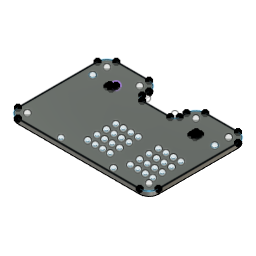
合页连接板-方案二-改 v3 (Autodesk Fusion 360 design; units mm, degrees)
Autodesk Fusion 360 part; units mm, degrees
sketch "草图1" plane through (0, 0, 0) normal (0, 0, 1) x (1, 0, 0)
  line L0 (75, -52.5) -> (-75, -52.5)
  line L1 (-75, -52.5) -> (-75, 52.5)
  line L2 (-75, 52.5) -> (75, 52.5)
  line L3 (75, 52.5) -> (75, -52.5)
  line L4 (75, -52.5) -> (-75, 52.5) construction
  line L5 (-75, -52.5) -> (75, 52.5) construction
  line L6 (-75, 27.5) -> (75, 27.5) construction
  line L7 (0, 52.5) -> (0, 0) construction
  line L8 (-35, 52.5) -> (-35, 27.5) construction
  line L9 (35, 52.5) -> (35, 27.5) construction
  circle A0 centre (-65.15, 27.5) radius 2.65
  circle A1 centre (65.15, 27.5) radius 2.65
  line L10 (-65.15, 30.15) -> (-65.15, 24.85) construction
  line L11 (65.15, 24.85) -> (65.15, 30.15) construction
  line L12 (65.15, 24.85) -> (-65.15, 24.85)
  line L13 (-65.15, 30.15) -> (65.15, 30.15)
  circle A2 centre (-46.85, 27.5) radius 2.65
  circle A3 centre (-42.85, 27.5) radius 2.65
  circle A4 centre (42.85, 27.5) radius 2.65
  circle A5 centre (46.85, 27.5) radius 2.65
  line L14 (-75, -5.5) -> (75, -5.5) construction
  line L15 (-75, -35.5) -> (75, -35.5) construction
  line L16 (-75, -47.5) -> (75, -47.5) construction
  circle A6 centre (-24, -47.5) radius 1.525
  circle A7 centre (32, -47.5) radius 1.525
  line L17 (-75, -25.5) -> (75, -25.5) construction
  line L18 (-75, -15.5) -> (75, -15.5) construction
  line L19 (62, -35.5) -> (62, -5.5) construction
  line L20 (-7.5, -35.5) -> (-7.5, -5.5) construction
  line L21 (0.5, -35.5) -> (0.5, -5.5) construction
  line L22 (8.5, -35.5) -> (8.5, -5.5) construction
  line L23 (16.5, -35.5) -> (16.5, -5.5) construction
  line L24 (38, -35.5) -> (38, -5.5) construction
  line L25 (46, -35.5) -> (46, -5.5) construction
  line L26 (54, -35.5) -> (54, -5.5) construction
  circle A8 centre (62, -5.5) radius 1.5
  circle A9 centre (62, -15.5) radius 1.5
  circle A10 centre (62, -25.5) radius 1.5
  circle A11 centre (62, -35.5) radius 1.5
  circle A12 centre (54, -5.5) radius 1.5
  circle A13 centre (54, -15.5) radius 1.5
  circle A14 centre (54, -25.5) radius 1.5
  circle A15 centre (54, -35.5) radius 1.5
  circle A16 centre (46, -5.5) radius 1.5
  circle A17 centre (46, -15.5) radius 1.5
  circle A18 centre (46, -25.5) radius 1.5
  circle A19 centre (38, -25.5) radius 1.5
  circle A20 centre (38, -5.5) radius 1.5
  circle A21 centre (38, -15.5) radius 1.5
  circle A22 centre (38, -35.5) radius 1.5
  circle A23 centre (46, -35.5) radius 1.5
  circle A24 centre (16.5, -5.5) radius 1.5
  circle A25 centre (8.5, -5.5) radius 1.5
  circle A26 centre (0.5, -5.5) radius 1.5
  circle A27 centre (-7.5, -5.5) radius 1.5
  circle A28 centre (16.5, -15.5) radius 1.5
  circle A29 centre (8.5, -15.5) radius 1.5
  circle A30 centre (0.5, -15.5) radius 1.5
  circle A31 centre (-7.5, -15.5) radius 1.5
  circle A32 centre (-7.5, -25.5) radius 1.5
  circle A33 centre (0.5, -25.5) radius 1.5
  circle A34 centre (8.5, -25.5) radius 1.5
  circle A35 centre (16.5, -25.5) radius 1.5
  circle A36 centre (16.5, -35.5) radius 1.5
  circle A37 centre (8.5, -35.5) radius 1.5
  circle A38 centre (0.5, -35.5) radius 1.5
  circle A39 centre (-7.5, -35.5) radius 1.5
  line L27 (-20, 52.5) -> (-20, 30.15)
  line L28 (20, 52.5) -> (20, 30.15)
  point P0 (-65.15, 27.5)
  point P1 (65.15, 27.5)
  point P2 (-44.85, 27.5)
  point P3 (44.85, 27.5)
  point P4 (0, 27.5)
  point P5 (-46.85, 27.5)
  point P6 (-42.85, 27.5)
  point P7 (42.85, 27.5)
  point P8 (46.85, 27.5)
  point P9 (32, -47.5)
  point P10 (-24, -47.5)
  point P11 (0.5, -35.5)
  point P12 (8.5, -35.5)
  point P13 (16.5, -35.5)
  point P14 (-7.5, -25.5)
  point P15 (-7.5, -5.5)
  point P16 (-7.5, -35.5)
  point P17 (-7.5, -15.5)
  point P18 (-7.5, -25.5)
  point P19 (62, -35.5)
  point P20 (62, -25.5)
  point P21 (62, -15.5)
  point P22 (62, -5.5)
  point P23 (54, -35.5)
  point P24 (46, -35.5)
  point P25 (38, -35.5)
  point P26 (0.5, -25.5)
  point P27 (0.5, -15.5)
  point P28 (0.5, -5.5)
  point P29 (8.5, -25.5)
  point P30 (8.5, -15.5)
  point P31 (8.5, -5.5)
  point P32 (16.5, -25.5)
  point P33 (16.5, -15.5)
  point P34 (16.5, -5.5)
  point P35 (38, -25.5)
  point P36 (38, -15.5)
  point P37 (38, -5.5)
  point P38 (46, -25.5)
  point P39 (46, -15.5)
  point P40 (46, -5.5)
  point P41 (54, -25.5)
  point P42 (54, -15.5)
  point P43 (54, -5.5)
  dimension "d1" = 150
  dimension "d2" = 105
  dimension "d3" = 25
  dimension "d4" = 20.3
  dimension "d5" = 20.3
  dimension "d6" = 9.85
  dimension "d7" = 44.85
  dimension "d8" = 9.85
  dimension "d9" = 44.85
  dimension "d10" = 40
  dimension "d11" = 40
  dimension "d12" = 70
  dimension "d13" = 5.3
  dimension "d14" = 5.3
  dimension "d15" = 2
  dimension "d16" = 2
  dimension "d17" = 2
  dimension "d18" = 2
  dimension "d20" = 30
  dimension "d24" = 56
  dimension "d25" = 3.05
  dimension "d26" = 3.05
  dimension "d27" = 10
  dimension "d28" = 10
  dimension "d29" = 10
  dimension "d30" = 13
  dimension "d35" = 8
  dimension "d36" = 16
  dimension "d37" = 24
  dimension "d38" = 3
  dimension "d39" = 3
  dimension "d40" = 3
  dimension "d41" = 3
  dimension "d42" = 3
  dimension "d43" = 3
  dimension "d44" = 3
  dimension "d45" = 3
  dimension "d46" = 3
  dimension "d47" = 3
  dimension "d48" = 3
  dimension "d49" = 3
  dimension "d50" = 3
  dimension "d51" = 3
  dimension "d52" = 3
  dimension "d53" = 3
  dimension "d54" = 3
  dimension "d55" = 3
  dimension "d56" = 3
  dimension "d57" = 3
  dimension "d58" = 3
  dimension "d59" = 3
  dimension "d60" = 3
  dimension "d61" = 3
  dimension "d62" = 3
  dimension "d63" = 3
  dimension "d64" = 3
  dimension "d65" = 3
  dimension "d66" = 3
  dimension "d67" = 3
  dimension "d68" = 3
  dimension "d69" = 3
  dimension "d72" = 21.5
  dimension "d73" = 21.5
  dimension "d74" = 8
  dimension "d75" = 8
  dimension "d76" = 8
  dimension "d77" = 20
  dimension "d84" = 51
  dimension "d87" = 5
  dimension "d88" = 12
  constraint horizontal L0
  constraint perpendicular L0 L1
  constraint parallel L0 L2
  constraint parallel L1 L3
  constraint coincident L4 L7.end
  constraint coincident L5 L7.end
  constraint coincident L7.end origin
  constraint coincident L1 L6.start
  constraint coincident L3 L6.end
  constraint perpendicular L3 L6
  constraint coincident L6 P0
  constraint coincident L6 P1
  constraint coincident L6 P2
  constraint coincident L6 P3
  constraint midpoint L2 L7.start
  constraint symmetric P2 P3 L7
  constraint midpoint L6 P4
  constraint coincident L2 L8.start
  constraint coincident L6 L8.end
  constraint perpendicular L6 L8
  constraint coincident L2 L9.start
  constraint coincident L6 L9.end
  constraint perpendicular L6 L9
  constraint coincident P0 A0.centre
  constraint coincident P1 A1.centre
  constraint coincident A0 L10.start
  constraint coincident A0 L10.end
  constraint perpendicular L6 L10
  constraint coincident A1 L11.start
  constraint coincident A1 L11.end
  constraint perpendicular L6 L11
  constraint tangent A0 L12
  constraint coincident L6 P5
  constraint coincident L6 P6
  constraint coincident L6 P7
  constraint coincident L6 P8
  constraint coincident P5 A2.centre
  constraint tangent L12 A2
  constraint coincident P6 A3.centre
  constraint tangent L12 A3
  constraint coincident P7 A4.centre
  constraint tangent L12 A4
  constraint coincident P8 A5.centre
  constraint tangent L12 A5
  constraint coincident L1 L14.start
  constraint coincident L3 L14.end
  constraint perpendicular L3 L14
  constraint coincident L1 L15.start
  constraint coincident L3 L15.end
  constraint perpendicular L3 L15
  constraint coincident L1 L16.start
  constraint coincident L3 L16.end
  constraint perpendicular L3 L16
  constraint coincident L16 P9
  constraint coincident L16 P10
  constraint coincident P10 A6.centre
  constraint coincident P9 A7.centre
  constraint coincident L1 L17.start
  constraint coincident L3 L17.end
  constraint perpendicular L3 L17
  constraint coincident L1 L18.start
  constraint coincident L3 L18.end
  constraint perpendicular L3 L18
  constraint coincident L15 P19
  constraint coincident L14 P22
  constraint perpendicular L14 L19
  constraint coincident L15 P16
  constraint coincident L14 P15
  constraint perpendicular L14 L20
  constraint coincident L15 P11
  constraint coincident L15 P12
  constraint coincident L15 P13
  constraint coincident L20 P18
  constraint coincident L17 P18
  constraint coincident P15 L20.end
  constraint coincident P16 L20.start
  constraint coincident L18 P17
  constraint coincident L20 P17
  constraint coincident P18 P14
  constraint coincident P19 L19.start
  constraint coincident L19 P20
  constraint coincident L17 P20
  constraint coincident L19 P21
  constraint coincident L18 P21
  constraint coincident P22 L19.end
  constraint coincident L15 P23
  constraint coincident L15 P24
  constraint coincident L15 P25
  constraint coincident L17 P26
  constraint coincident L18 P27
  constraint coincident L14 P28
  constraint coincident L17 P29
  constraint coincident L18 P30
  constraint coincident L14 P31
  constraint coincident L17 P32
  constraint coincident L18 P33
  constraint coincident L14 P34
  constraint coincident L17 P35
  constraint coincident L18 P36
  constraint coincident L14 P37
  constraint coincident L17 P38
  constraint coincident L18 P39
  constraint coincident L14 P40
  constraint coincident L17 P41
  constraint coincident L18 P42
  constraint coincident L14 P43
  constraint coincident P11 L21.start
  constraint coincident P28 L21.end
  constraint perpendicular L14 L21
  constraint coincident P12 L22.start
  constraint coincident P31 L22.end
  constraint perpendicular L14 L22
  constraint coincident P13 L23.start
  constraint coincident P34 L23.end
  constraint perpendicular L14 L23
  constraint coincident P25 L24.start
  constraint coincident P37 L24.end
  constraint perpendicular L14 L24
  constraint coincident P24 L25.start
  constraint coincident P40 L25.end
  constraint perpendicular L14 L25
  constraint coincident P23 L26.start
  constraint coincident P43 L26.end
  constraint perpendicular L14 L26
  constraint coincident P21 A9.centre
  constraint coincident P20 A10.centre
  constraint coincident P42 A13.centre
  constraint coincident P41 A14.centre
  constraint coincident P39 A17.centre
  constraint coincident P38 A18.centre
  constraint coincident P35 A19.centre
  constraint coincident P36 A21.centre
  constraint coincident P33 A28.centre
  constraint coincident P30 A29.centre
  constraint coincident P27 A30.centre
  constraint coincident P17 A31.centre
  constraint coincident P26 A33.centre
  constraint coincident P29 A34.centre
  constraint coincident P32 A35.centre
  constraint coincident P42 L26
  constraint coincident L26 P41
  constraint coincident P38 L25
  constraint coincident P39 L25
  constraint coincident P36 L24
  constraint coincident L24 P35
  constraint coincident L23 P33
  constraint coincident P30 L22
  constraint coincident L22 P29
  constraint coincident L21 P26
  constraint coincident P27 L21
  constraint coincident L2 L27.start
  constraint coincident L13 L27.end
  constraint perpendicular L13 L27
  constraint coincident L2 L28.start
  constraint coincident L13 L28.end
  constraint perpendicular L13 L28
  measures "d1" distance of L1.end L2.end
  measures "d2" distance of L0.end L1.end
  measures "d3" distance of L2 L6
  measures "d4" distance of P0 P2
  measures "d5" distance of P1 P3
  measures "d6" distance of L1 P0
  measures "d7" distance of P2 P4
  measures "d8" distance of L6.end P1
  measures "d9" distance of P3 P4
  measures "d10" distance of L1 L8
  measures "d11" distance of L3 L9
  measures "d12" distance of L8.end L9.end
  measures "d13" diameter of A0
  measures "d14" diameter of A1
  measures "d15" distance of P2 P5
  measures "d16" distance of P2 P6
  measures "d17" distance of P3 P7
  measures "d18" distance of P3 P8
  measures "d20" distance of L14 L15
  measures "d24" distance of P9 P10
  measures "d25" diameter of A6
  measures "d26" diameter of A7
  measures "d27" distance of L14 L18
  measures "d28" distance of L15 L17
  measures "d29" distance of L17 L18
  measures "d30" distance of L3 L19
  measures "d35" distance of P19 P23
  measures "d36" distance of P19 P24
  measures "d37" distance of L19 P25
  measures "d38" diameter of A8
  measures "d39" diameter of A9
  measures "d40" diameter of A10
  measures "d41" diameter of A11
  measures "d42" diameter of A12
  measures "d43" diameter of A13
  measures "d44" diameter of A14
  measures "d45" diameter of A15
  measures "d46" diameter of A16
  measures "d47" diameter of A17
  measures "d48" diameter of A18
  measures "d49" diameter of A19
  measures "d50" diameter of A20
  measures "d51" diameter of A21
  measures "d52" diameter of A22
  measures "d53" diameter of A23
  measures "d54" diameter of A24
  measures "d55" diameter of A25
  measures "d56" diameter of A26
  measures "d57" diameter of A27
  measures "d58" diameter of A28
  measures "d59" diameter of A29
  measures "d60" diameter of A30
  measures "d61" diameter of A31
  measures "d62" diameter of A32
  measures "d63" diameter of A33
  measures "d64" diameter of A34
  measures "d65" diameter of A35
  measures "d66" diameter of A36
  measures "d67" diameter of A37
  measures "d68" diameter of A38
  measures "d69" diameter of A39
  measures "d72" distance of P35 P32
  measures "d73" distance of P33 P36
  measures "d74" distance of L22 L23
  measures "d75" distance of L21 L22
  measures "d76" distance of L20 L21
  measures "d77" distance of L7 L27
  measures "d84" distance of L1 P10
  measures "d87" distance of L0 L16
  measures "d88" distance of L15 L16
extrude "拉伸4" add sketch "草图1" along normal blind 5 contours L0 L1 L2 L3 A0 A1 L12 L13 L27 L28 | L12 L13 A3 A4 | A1 L12 L13 A5 | A0 L12 L13 A2
fillet "圆角3" radius 10 6 edges at (-75, 52.5, 2.5) (-75, -52.5, 2.5) (75, -52.5, 2.5) (-20, 52.5, 2.5) (75, 52.5, 2.5) (20, 52.5, 2.5)
fillet "圆角4" radius 5 2 edges at (-20, 30.15, 2.5) (20, 30.15, 2.5)
sketch "草图2" plane through (0, 0, 5) normal (0, 0, 1) x (-1, 0, 0)
  arc A0 (-30, -52.5) -> (-20, -42.5) centre (-30, -42.5) ccw
  line L0 (-20, -42.5) -> (-20, -35.15)
  arc A1 (-15, -30.15) -> (-20, -35.15) centre (-15, -35.15) ccw
  line L1 (-15, -30.15) -> (15, -30.15)
  arc A2 (20, -35.15) -> (15, -30.15) centre (15, -35.15) ccw
  line L2 (20, -35.15) -> (20, -42.5)
  arc A3 (20, -42.5) -> (30, -52.5) centre (30, -42.5) ccw
  line L3 (30, -52.5) -> (65, -52.5)
  arc A4 (65, -52.5) -> (75, -42.5) centre (65, -42.5) ccw
  line L4 (75, -42.5) -> (75, 42.5)
  arc A5 (75, 42.5) -> (65, 52.5) centre (65, 42.5) ccw
  line L5 (65, 52.5) -> (-65, 52.5)
  arc A6 (-65, 52.5) -> (-75, 42.5) centre (-65, 42.5) ccw
  line L6 (-75, 42.5) -> (-75, -42.5)
  arc A7 (-75, -42.5) -> (-65, -52.5) centre (-65, -42.5) ccw
  line L7 (-65, -52.5) -> (-30, -52.5)
  circle A8 centre (7.5, 15.5) radius 1.5
  circle A9 centre (7.5, 25.5) radius 1.5
  circle A10 centre (-8.5, 25.5) radius 1.5
  circle A11 centre (-0.5, 25.5) radius 1.5
  arc A12 (46.85, -30.15) -> (46.85, -24.85) centre (46.85, -27.5) ccw
  line L8 (46.85, -30.15) -> (42.85, -30.15)
  arc A13 (42.85, -24.85) -> (42.85, -30.15) centre (42.85, -27.5) ccw
  line L9 (42.85, -24.85) -> (46.85, -24.85)
  circle A14 centre (65.15, -27.5) radius 2.65
  arc A15 (-42.85, -30.15) -> (-42.85, -24.85) centre (-42.85, -27.5) ccw
  line L10 (-42.85, -30.15) -> (-46.85, -30.15)
  arc A16 (-46.85, -24.85) -> (-46.85, -30.15) centre (-46.85, -27.5) ccw
  line L11 (-46.85, -24.85) -> (-42.85, -24.85)
  circle A17 centre (-0.5, 35.5) radius 1.5
  circle A18 centre (-16.5, 25.5) radius 1.5
  circle A19 centre (-16.5, 35.5) radius 1.5
  circle A20 centre (-8.5, 35.5) radius 1.5
  circle A21 centre (-65.15, -27.5) radius 2.65
  circle A22 centre (7.5, 35.5) radius 1.5
  circle A23 centre (-0.5, 15.5) radius 1.5
  circle A24 centre (-8.5, 15.5) radius 1.5
  circle A25 centre (-16.5, 15.5) radius 1.5
  circle A26 centre (7.5, 5.5) radius 1.5
  circle A27 centre (-0.5, 5.5) radius 1.5
  circle A28 centre (-8.5, 5.5) radius 1.5
  circle A29 centre (-16.5, 5.5) radius 1.5
  circle A30 centre (-46, 35.5) radius 1.5
  circle A31 centre (-38, 35.5) radius 1.5
  circle A32 centre (-38, 15.5) radius 1.5
  circle A33 centre (-38, 5.5) radius 1.5
  circle A34 centre (-38, 25.5) radius 1.5
  circle A35 centre (-46, 25.5) radius 1.5
  circle A36 centre (-46, 15.5) radius 1.5
  circle A37 centre (-46, 5.5) radius 1.5
  circle A38 centre (-54, 35.5) radius 1.5
  circle A39 centre (-54, 25.5) radius 1.5
  circle A40 centre (-54, 15.5) radius 1.5
  circle A41 centre (-54, 5.5) radius 1.5
  circle A42 centre (-62, 35.5) radius 1.5
  circle A43 centre (-62, 25.5) radius 1.5
  circle A44 centre (-62, 15.5) radius 1.5
  circle A45 centre (-62, 5.5) radius 1.5
  circle A46 centre (-32, 47.5) radius 1.525
  circle A47 centre (24, 47.5) radius 1.525
  circle A48 centre (-32, 47.5) radius 1.525
  circle A49 centre (24, 47.5) radius 1.525
  circle A50 centre (7.5, 35.5) radius 1.5
  circle A51 centre (-0.5, 35.5) radius 1.5
  circle A52 centre (-8.5, 35.5) radius 1.5
  circle A53 centre (-16.5, 35.5) radius 1.5
  circle A54 centre (-38, 35.5) radius 1.5
  circle A55 centre (-46, 35.5) radius 1.5
  circle A56 centre (-54, 35.5) radius 1.5
  circle A57 centre (-62, 35.5) radius 1.5
  circle A58 centre (-62, 25.5) radius 1.5
  circle A59 centre (-54, 25.5) radius 1.5
  circle A60 centre (-46, 25.5) radius 1.5
  circle A61 centre (-38, 25.5) radius 1.5
  circle A62 centre (-16.5, 25.5) radius 1.5
  circle A63 centre (-8.5, 25.5) radius 1.5
  circle A64 centre (-0.5, 25.5) radius 1.5
  circle A65 centre (7.5, 25.5) radius 1.5
  circle A66 centre (7.5, 15.5) radius 1.5
  circle A67 centre (-0.5, 15.5) radius 1.5
  circle A68 centre (-8.5, 15.5) radius 1.5
  circle A69 centre (-16.5, 15.5) radius 1.5
  circle A70 centre (-38, 15.5) radius 1.5
  circle A71 centre (-46, 15.5) radius 1.5
  circle A72 centre (-54, 15.5) radius 1.5
  circle A73 centre (-62, 15.5) radius 1.5
  circle A74 centre (-62, 5.5) radius 1.5
  circle A75 centre (-54, 5.5) radius 1.5
  circle A76 centre (-46, 5.5) radius 1.5
  circle A77 centre (-38, 5.5) radius 1.5
  circle A78 centre (-16.5, 5.5) radius 1.5
  circle A79 centre (-8.5, 5.5) radius 1.5
  circle A80 centre (-0.5, 5.5) radius 1.5
  circle A81 centre (7.5, 5.5) radius 1.5
  circle A82 centre (65.15, -27.5) radius 2.65
  circle A83 centre (-65.15, -27.5) radius 2.65
  line L12 (-46.85, -24.85) -> (-42.85, -24.85)
  line L13 (-46.85, -30.15) -> (-42.85, -30.15)
  arc A84 (-46.85, -24.85) -> (-46.85, -30.15) centre (-46.85, -27.5) ccw
  arc A85 (-42.85, -30.15) -> (-42.85, -24.85) centre (-42.85, -27.5) ccw
  arc A86 (42.85, -24.85) -> (42.85, -30.15) centre (42.85, -27.5) ccw
  arc A87 (46.85, -30.15) -> (46.85, -24.85) centre (46.85, -27.5) ccw
  line L14 (42.85, -24.85) -> (46.85, -24.85)
  line L15 (42.85, -30.15) -> (46.85, -30.15)
  line L16 (-65, -52.5) -> (-30, -52.5)
  line L17 (-20, -42.5) -> (-20, -35.15)
  line L18 (20, -35.15) -> (20, -42.5)
  line L19 (15, -30.15) -> (-15, -30.15)
  line L20 (30, -52.5) -> (65, -52.5)
  line L21 (-75, -42.5) -> (-75, 42.5)
  line L22 (-65, 52.5) -> (65, 52.5)
  line L23 (75, 42.5) -> (75, -42.5)
  arc A88 (-65, 52.5) -> (-75, 42.5) centre (-65, 42.5) ccw
  arc A89 (75, 42.5) -> (65, 52.5) centre (65, 42.5) ccw
  arc A90 (65, -52.5) -> (75, -42.5) centre (65, -42.5) ccw
  arc A91 (20, -42.5) -> (30, -52.5) centre (30, -42.5) ccw
  arc A92 (20, -35.15) -> (15, -30.15) centre (15, -35.15) ccw
  arc A93 (-15, -30.15) -> (-20, -35.15) centre (-15, -35.15) ccw
  arc A94 (-30, -52.5) -> (-20, -42.5) centre (-30, -42.5) ccw
  arc A95 (-75, -42.5) -> (-65, -52.5) centre (-65, -42.5) ccw
  dimension "d95" = 21.5
  constraint concentric A46 A48
  constraint concentric A47 A49
  constraint concentric A22 A50
  constraint concentric A17 A51
  constraint concentric A20 A52
  constraint concentric A19 A53
  constraint concentric A31 A54
  constraint concentric A30 A55
  constraint concentric A38 A56
  constraint concentric A42 A57
  constraint concentric A43 A58
  constraint concentric A39 A59
  constraint concentric A35 A60
  constraint concentric A34 A61
  constraint concentric A18 A62
  constraint concentric A10 A63
  constraint concentric A11 A64
  constraint concentric A9 A65
  constraint concentric A8 A66
  constraint concentric A23 A67
  constraint concentric A24 A68
  constraint concentric A25 A69
  constraint concentric A32 A70
  constraint concentric A36 A71
  constraint concentric A40 A72
  constraint concentric A44 A73
  constraint concentric A45 A74
  constraint concentric A41 A75
  constraint concentric A37 A76
  constraint concentric A33 A77
  constraint concentric A29 A78
  constraint concentric A28 A79
  constraint concentric A27 A80
  constraint concentric A26 A81
  constraint concentric A14 A82
  constraint concentric A21 A83
  constraint coincident A16.start L11.start
  constraint coincident A15.end L11.end
  constraint coincident L10.end A16.end
  constraint coincident A15.start L10.start
  constraint coincident A16.centre A84.centre
  constraint coincident A15.centre A85.centre
  constraint coincident L8.end A13.end
  constraint coincident A13.start L9.start
  constraint coincident A13.centre A86.centre
  constraint coincident A12.end L9.end
  constraint coincident A12.centre A87.centre
  constraint tangent A12 L15
  constraint coincident A7.end L7.start
  constraint coincident A0.start L7.end
  constraint coincident A0.end L0.start
  constraint coincident L0.end A1.end
  constraint coincident A2.start L2.start
  constraint coincident L2.end A3.start
  constraint coincident L1.end A2.end
  constraint coincident A1.start L1.start
  constraint coincident A3.end L3.start
  constraint coincident L3.end A4.start
  constraint coincident L6.end A7.start
  constraint coincident A6.end L6.start
  constraint coincident L5.end A6.start
  constraint coincident A5.end L5.start
  constraint coincident L4.end A5.start
  constraint coincident A4.end L4.start
  measures "d95" distance of A18.centre A34.centre
extrude "拉伸3" [suppressed]
extrude "拉伸2" [suppressed]
fillet "圆角1" [suppressed]
fillet "圆角2" [suppressed]
extrude "拉伸1" [suppressed]
